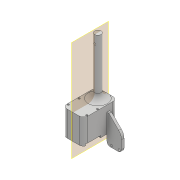
# Autodesk Inventor part: core_attachment
Saved by Autodesk Inventor 2018 (Build 220112000, 112)
## iProperties
Created: 2018-05-21
Part Number: core_attachment
Material: Generic
Document SubType Name: Modeling
Designer: Bardo91
Density: 1 g/cm^3
Appearance: Default
Author: Bardo91
Autodesk Inventor part; units mm, degrees
ref_plane "XZ Plane" through (0, 0, 0) normal (0, 1, 0) x (-1, 0, 0)
ref_plane "XY Plane" through (0, 0, 0) normal (0, 0, 1) x (1, 0, 0)
sketch "Sketch1" plane through (0, 0, 0) normal (0, 0, 1) x (1, 0, 0)
  line L0 (0, 0) -> (25, 0)
  line L1 (25, 0) -> (25, 45.5)
  line L2 (25, 45.5) -> (0, 45.5)
  line L3 (0, 45.5) -> (0, 0)
  line L4 (-4, 49.5) -> (29, 49.5)
  line L5 (29, 49.5) -> (29, -4)
  line L6 (29, -4) -> (-4, -4)
  line L7 (-4, -4) -> (-4, 49.5)
  dimension "d0" = 25
  dimension "d1" = 45.5
  dimension "d2" = 4
  constraints: 16 end point, 6 perpendicular, 1 horizontal, 3 other
  measures "d0" distance of L0.start L0.end
  measures "d1" distance of L0.end L1.end
  measures "d2" distance between parallel lines of L2 L4
extrude "Extrusion1" add sketch "Sketch1" along normal blind 40 contours L3 L2 L1 L0 | L4 L5 L6 L7
extrude "Extrusion2" cut sketch "Sketch1" along normal blind 38 contours L3 L2 L1 L0
sketch "Sketch2" plane through (29, -4, 0) normal (1, 0, 0) x (0, 0, -1)
  line L0 (0, 4) -> (-3, 4)
  line L1 (0, 4) -> (-38, 4) projected
  line L2 (-3, 4) -> (-3, 27)
  line L3 (-3, 27) -> (0, 27)
  line L4 (0, 27) -> (0, 4)
  line L5 (0, 0) -> (0, 53.5) projected
  dimension "d7" = 3
  dimension "d8" = 23
  constraints: 8 end point, 2 perpendicular, 1 collinear, 1 point on line
  measures "d7" distance of L0.start L0.end
  measures "d8" distance of L0.end L2.end
extrude "Extrusion3" cut sketch "Sketch2" against normal through all
sketch "Sketch3" plane through (0, 0, 40) normal (0, 0, 1) x (1, 0, 0)
  line L0 (-4, 49.5) -> (29, 49.5) projected
  line L1 (12.5, 49.5) -> (12.5, 45.5)
  line L2 (25, 45.5) -> (0, 45.5) projected
  line L3 (12.5, 45.5) -> (12.5, 35.2)
  circle A0 centre (12.5, 35.2) radius 5
  point P0 (0, 0)
  dimension "d11" = 10.3
  dimension "d12" = 10
  constraints: 4 end point, 2 midpoint, 1 centre point, 1 coincident, 1 point on line
  measures "d11" distance of L1.end L3.end
  measures "d12" diameter of A0
extrude "Extrusion4" add sketch "Sketch3" along normal blind 90
fillet "Fillet1" radius 10 1 edges at (7.5, 35.2, 40)
sketch "Sketch4" plane through (-4, 49.5, 0) normal (0, 1, 0) x (1, 0, 0)
  line L0 (11.5, -130) -> (21.5, -130) projected
  line L1 (16.5, -130) -> (16.5, -117)
  circle A0 centre (16.5, -117) radius 1.5
  point P0 (4, 0)
  dimension "d16" = 13
  dimension "d17" = 3
  constraints: 2 end point, 1 centre point, 1 coincident, 1 midpoint, 1 vertical
  measures "d16" distance of L1.start L1.end
  measures "d17" diameter of A0
extrude "Extrusion5" cut sketch "Sketch4" against normal through all
fillet "Fillet2" radius 7 4 edges at (29, -4, 20) (29, 49.5, 20) (-4, 49.5, 20) (-4, -4, 20)
sketch "Sketch5" plane through (29, 23, 3) normal (0, 0, -1) x (-1, 0, 0)
  line L0 (0, 0) -> (4, 0) projected
  line L1 (2, 0) -> (2, -3)
  line L2 (2, -23) -> (2, -20)
  line L3 (29, 0) -> (33, 0) projected
  line L4 (31, 0) -> (31, -3)
  line L5 (31, -23) -> (31, -20)
  circle A0 centre (2, -20) radius 1.4
  circle A1 centre (2, -3) radius 1.4
  circle A2 centre (31, -3) radius 1.4
  circle A3 centre (31, -20) radius 1.4
  point P0 (29, -23)
  dimension "d21" = 3
  dimension "d22" = 3
  dimension "d23" = 3
  dimension "d24" = 3
  dimension "d25" = 2.8
  dimension "d26" = 2.8
  dimension "d27" = 2.8
  dimension "d28" = 2.8
  constraints: 8 end point, 4 centre point, 4 coincident, 4 vertical, 2 midpoint
  measures "d21" distance of L1.start L1.end
  measures "d22" distance of L2.start L2.end
  measures "d23" distance of L4.start L4.end
  measures "d24" distance of L5.start L5.end
  measures "d25" diameter of A0
  measures "d26" diameter of A1
  measures "d27" diameter of A2
  measures "d28" diameter of A3
extrude "Extrusion6" cut sketch "Sketch5" against normal through all
sketch "Sketch6" plane through (-4, 23, 0) normal (-1, 0, 0) x (0, 0, 1)
  line L0 (50, 17.2) -> (50, 7.2) projected
  line L1 (50, 12.2) -> (0, 12.2)
  line L2 (0, 12.2) -> (0, 14.2)
  line L3 (0, 14.2) -> (30, 14.2)
  line L4 (30, 14.2) -> (30, 10.2)
  line L5 (30, 10.2) -> (0, 10.2)
  line L6 (0, 0) -> (0, 19.5) projected
  line L7 (0, 10.2) -> (0, 12.2)
  point P0 (0, -23)
  dimension "d31" = 2
  dimension "d32" = 30
  dimension "d33" = 4
  constraints: 12 end point, 3 horizontal, 3 perpendicular, 1 midpoint, 1 point on line
  measures "d31" distance of L1.end L2.end
  measures "d32" distance of L2.end L3.end
  measures "d33" distance of L3.end L4.end
extrude "Extrusion7" add sketch "Sketch6" along normal blind 23
chamfer "Chamfer1" distance 20 angle 45 1 edges at (-27, 35.2, 30)
sketch "Sketch7" plane through (0, 0, 0) normal (0, 0, -1) x (-1, 0, 0)
  line L0 (27, 37.2) -> (27, 33.2) projected
  line L1 (4, 37.2) -> (4, 33.2) projected
  line L2 (27, 37.2) -> (4, 37.2)
  line L3 (4, 37.2) -> (4, 33.2)
  line L4 (4, 33.2) -> (27, 33.2)
  line L5 (27, 33.2) -> (27, 37.2)
  point P0 (0, 0)
  constraints: 8 end point, 2 parallel, 1 horizontal, 1 perpendicular
extrude "Extrusion8" add sketch "Sketch7" along normal blind 15
fillet "Fillet3" radius 5 2 edges at (-4, 35.2, -15) (-27, 35.2, -15)
sketch "Sketch8" plane through (-4, 33.2, 0) normal (0, -1, 0) x (1, 0, 0)
  line L0 (-5, -15) -> (-18, -15) projected
  line L1 (-11.5, -15) -> (-11.5, -12)
  line L2 (-11.5, -12) -> (-19.5, -12)
  line L3 (-11.5, -12) -> (-7.5, -12)
  circle A0 centre (-19.5, -12) radius 1.5
  circle A1 centre (-7.5, -12) radius 1.5
  point P0 (4, 0)
  dimension "d42" = 3
  dimension "d43" = 8
  dimension "d44" = 4
  dimension "d45" = 3
  dimension "d46" = 3
  constraints: 6 end point, 2 centre point, 2 coincident, 1 horizontal, 1 midpoint, 1 perpendicular, 1 vertical
  measures "d42" distance of L1.start L1.end
  measures "d43" distance of L1.end L2.end
  measures "d44" distance of L1.end L3.end
  measures "d45" diameter of A0
  measures "d46" diameter of A1
extrude "Extrusion9" cut sketch "Sketch8" against normal through all
fillet "Fillet4" radius 15 1 edges at (-27, 35.2, 10)
ref_plane "Work Plane1" through (12.5, 0, 0) normal (1, 0, 0) x (0, 1, 0)
mirror "Mirror1" about plane through (12.5, 0, 0) normal (1, 0, 0) of "Extrusion7", "Chamfer1", "Extrusion8", "Fillet3", "Extrusion9", "Fillet4"
equation "\"d25\" = d26"
equation "\"d27\" = d26"
equation "\"d28\" = d26"
body "Solid1"
